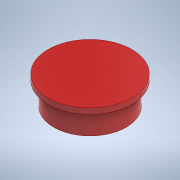
# Autodesk Inventor part: CapForSvBonyPlosse-40mm
Saved by Autodesk Inventor 2021.1 (Build 251245010, 245A)
## iProperties
Created: 2020-10-08
Part Number: CapForSvBonyPlosse-40mm
Material: PC/ABS Plastic
Document SubType Name: Modeling
Designer: robst
Density: 0.357273 g/cm^3
Appearance: Red
Author: robst
Autodesk Inventor part; units mm, degrees
ref_plane "YZ Plane" through (0, 0, 0) normal (1, 0, 0) x (0, 1, 0)
ref_plane "XZ Plane" through (0, 0, 0) normal (0, 1, 0) x (-1, 0, 0)
ref_plane "XY Plane" through (0, 0, 0) normal (0, 0, 1) x (1, 0, 0)
sketch "Sketch7" plane through (0, 0, 0) normal (0, 0, 1) x (1, 0, 0)
  line L0 (0, 0) -> (20.3518, 0)
  line L1 (20.3518, 0) -> (20.3517, 12.7)
  line L2 (20.3517, 12.7) -> (23.5267, 12.7)
  line L3 (23.5267, 12.7) -> (23.5267, 15.875)
  line L4 (23.5267, 15.875) -> (0, 15.875)
  line L5 (20.3518, 0) -> (17.1768, 0)
  line L6 (17.1768, 0) -> (17.1768, 12.7)
  line L7 (17.1768, 12.7) -> (0, 12.7)
  line L8 (0, 15.875) -> (0, 12.7)
  line L9 (0, -8.253) -> (0, 19.8963) projected
  dimension "d71" = 3.175
  dimension "d72" = 12.7
  dimension "d73" = 20.3517
  dimension "d77" = 3.175
  dimension "d78" = 3.175
  constraints: 18 end point, 5 perpendicular, 2 vertical, 1 horizontal, 1 point on line
  measures "d71" distance between parallel lines of L4 L2
  measures "d72" distance from line of L2 L0.start
  measures "d73" distance of L0.start L0.end
  measures "d77" distance of L2.end L1.end
  measures "d78" distance between parallel lines of L1 L6
revolve "Revolution3" add sketch "Sketch7" angle 360 about axis through (0, -10, 0) along (0, 1, 0) contours L6 L7 L8 L4 L3 L2 L1 L0
equation "\"d71\" = wallThickness"
equation "\"d72\" = caseHeightAboveLens"
equation "\"d73\" = a2MajorRadiusMax"
equation "\"d77\" = wallThickness"
equation "\"d78\" = wallThickness"
equation "\"baseDiameter\" = 31.75"
equation "\"baseRadius\" = 0.5 * baseDiameter"
equation "\"baseHeight\" = 25.4"
equation "\"middleDiameter\" = 34.29"
equation "\"middleRadius\" = 0.5 * middleDiameter"
equation "\"middleTopDiameter\" = 34.798"
equation "\"middleTopRadius\" = 0.5 * middleTopDiameter"
equation "\"middleHeight\" = 18.542"
equation "\"middleTopHeight\" = 30.734"
equation "\"topBaseDiameter\" = 34.798"
equation "\"topHeightDiameter\" = 40.894"
equation "\"topBaseRadius\" = 0.5 * topBaseDiameter"
equation "\"topHeightRadius\" = 0.5 * topHeightDiameter"
equation "\"topHeight\" = 7.62"
equation "\"d9\" = caseBottomThickness"
equation "\"wallThickness\" = 3.175"
equation "\"caseBottomThickness\" = 4.7625"
equation "\"caseHeightAboveLens\" = 12.7"
equation "\"baseWallThickness\" = 2.032"
equation "\"baseInteriorHeight\" = 15.24"
equation "\"interiorDiameter\" = 41.275"
equation "\"interiorRadius\" = 0.5 * interiorDiameter"
equation "\"outsideRadius\" = interiorRadius + wallThickness"
equation "\"outsideDiameter\" = 2 * outsideRadius"
equation "\"textRingDiameter\" = 0.75 * outsideDiameter"
equation "\"b2MajorDiameterMax\" = 41.275"
equation "\"b2MajorRadiusMax\" = 0.5 * b2MajorDiameterMax"
equation "\"b2MinorDiameterMax\" = 38.92042"
equation "\"b2MinorRadiusMax\" = 0.5 * b2MinorDiameterMax"
equation "\"b2MajorDiameterMin\" = 41.275"
equation "\"b2MajorRadiusMin\" = 0.5 * b2MajorDiameterMin"
equation "\"a2MinorDiameterMin\" = 37.66312"
equation "\"a2MinorRadiusMin\" = 0.5 * a2MinorDiameterMin"
equation "\"a2MajorDiameterMax\" = 40.7035"
equation "\"a2MajorRadiusMax\" = 0.5 * a2MajorDiameterMax"
body "Solid3"
